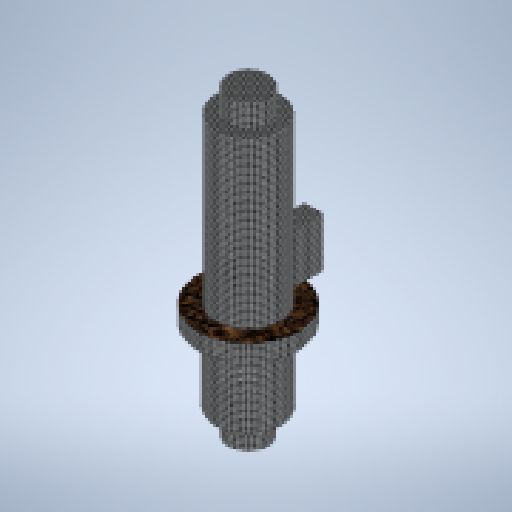
# Autodesk Inventor part: eje
Saved by Autodesk Inventor 2023 (Build 270158000, 158)
## iProperties
Created: 2024-07-31
Part Number: eje
Material: Generic
Document SubType Name: Modeling
Designer: sebas
Density: 1 g/cm^3
Appearance: Chrome - Polished
Author: sebas
Autodesk Inventor part; units mm, degrees
ref_plane "YZ Plane" through (0, 0, 0) normal (1, 0, 0) x (0, 1, 0)
ref_plane "XZ Plane" through (0, 0, 0) normal (0, 1, 0) x (-1, 0, 0)
ref_plane "XY Plane" through (0, 0, 0) normal (0, 0, 1) x (1, 0, 0)
sketch "Sketch1" plane through (0, 0, 0) normal (0, 1, 0) x (-1, 0, 0)
  circle A0 centre (0, 0) radius 12
  dimension "d0" = 24
  constraints: 1 centre point, 1 coincident
  measures "d0" diameter of A0
extrude "Extrusion1" add sketch "Sketch1" along normal blind 11
sketch "Sketch2" plane through (0, 11, 0) normal (0, 1, 0) x (1, 0, 0)
  circle A0 centre (0, 0) radius 15
  dimension "d3" = 30
  constraints: 1 centre point, 1 coincident
  measures "d3" diameter of A0
extrude "Extrusion2" add sketch "Sketch2" along normal blind 4
sketch "Sketch3" plane through (0, 15, 0) normal (0, 1, 0) x (1, 0, 0)
  circle A0 centre (0, 0) radius 20
  dimension "d6" = 40
  constraints: 1 centre point, 1 coincident
  measures "d6" diameter of A0
extrude "Extrusion3" add sketch "Sketch3" along normal blind 54
sketch "Sketch6" plane through (0, 69, 0) normal (0, 1, 0) x (1, 0, 0)
  circle A0 centre (0, 0) radius 30
  dimension "d15" = 60
  constraints: 1 centre point, 1 coincident
  measures "d15" diameter of A0
extrude "Extrusion6" add sketch "Sketch6" against normal blind 10
sketch "Sketch7" plane through (0, 69, 0) normal (0, 1, 0) x (1, 0, 0)
  arc A0 (-5.7, 18.6483) -> (5.7, 18.6483) centre (0, 0) ccw
  arc A1 (5.7, 19.1706) -> (-5.7, 19.1706) centre (0, 0) ccw
  circle A2 centre (0, 0) radius 20 projected
  line L0 (0, 20) -> (5.7, 20)
  line L1 (5.7, 20) -> (5.7, 39.5)
  line L2 (5.7, 39.5) -> (-5.7, 39.5)
  line L3 (-5.7, 39.5) -> (-5.7, 18.6483)
  line L4 (5.7, 18.6483) -> (5.7, 20)
  dimension "d18" = 39
  dimension "d19" = 40
  dimension "d20" = 5.7
  dimension "d21" = 19.5
  dimension "d22" = 11.4
  constraints: 10 end point, 4 point on circle, 3 horizontal, 2 centre point, 2 coincident, 2 perpendicular, 2 point on line, 1 collinear, 1 vertical alignment, 1 other
  measures "d18" diameter of A0
  measures "d19" diameter of A1
  measures "d20" distance of L0.start L0.end
  measures "d21" distance of L0.end L1.end
  measures "d22" distance of L1.end L2.end
extrude "Extrusion7" add sketch "Sketch7" along normal blind 30 contours L3 A1 L4 A0 | L3 L2 L1 L0 A1 | A1 L0 L4
sketch "Sketch8" plane through (0, 99, 0) normal (0, 1, 0) x (1, 0, 0)
  circle A0 centre (0, 0) radius 14.625
  circle A1 centre (0, 0) radius 15 projected
  circle A2 centre (0, 0) radius 19.5
  dimension "d27" = 39
  constraints: 2 centre point, 2 coincident
  measures "d27" diameter of A2
extrude "Extrusion8" add sketch "Sketch8" along normal blind 69.5 contours A0 | A1 | A2
sketch "Sketch9" plane through (0, 168.5, 0) normal (0, 1, 0) x (1, 0, 0)
  circle A0 centre (0, 0) radius 12.25
  dimension "d28" = 24.5
  constraints: 1 centre point, 1 coincident
  measures "d28" diameter of A0
extrude "Extrusion9" add sketch "Sketch9" along normal blind 14
body "Solid1"
